Links  big screw 6 printed_v1 (Autodesk Fusion 360 design; units mm, degrees)
Autodesk Fusion 360 part; units mm, degrees
note: some values were not read from the file. Chosen so that the rebuilt part matches the saved one: which face or edge a step refers to. Set by a fixed rule: which sketch regions a step uses.
sketch "passive link sketch" plane through (0, 0, 0) normal (0, 0, 1) x (1, 0, 0)
  line L0 (-16.4533, 8) -> (-16.4533, -8) construction
  line L1 (16.4533, -8) -> (16.4533, 8) construction
  line L2 (16.4533, 8) -> (-16.4533, -8) construction
  line L3 (-16.4533, 8) -> (16.4533, -8) construction
  circle A0 centre (12.5, 0) radius 4.5
  circle A1 centre (12.5, 0) radius 2.975
  circle A2 centre (12.5, 0) radius 8
  line L4 (0, 8) -> (0, -15) construction
  line L5 (12.5, 8) -> (0, 8)
  line L6 (0, -8) -> (12.5, -8)
  line L7 (12.5, -8) -> (12.5, 8)
  line L8 (12.5, 8) -> (-12.5, -8) construction
  line L9 (-12.5, 8) -> (12.5, -8) construction
  line L10 (16.4533, 8) -> (0, 8) construction
  line L11 (-12.5, 8) -> (-16.4533, 8) construction
  line L12 (-16.4533, -8) -> (-12.5, -8) construction
  line L13 (0, -8) -> (16.4533, -8) construction
  line L14 (0, -8) -> (-16.4533, -8) construction
  line L15 (-12.5, -8) -> (-12.5, 8)
  line L16 (-16.4533, 8) -> (0, 8) construction
  circle A3 centre (-12.5, 0) radius 8
  circle A4 centre (-12.5, 0) radius 2.975
  circle A5 centre (-12.5, 0) radius 4.5
  line L17 (0, -8) -> (-12.5, -8)
  line L18 (-12.5, 8) -> (0, 8)
  dimension "d2" = 16
  dimension "d3" = 9
  dimension "d4" = 5.95
  dimension "d5" = 16
  dimension "d6" = 12.5
  dimension "d7" = 25
  constraint horizontal L10
  constraint perpendicular L0 L10
  constraint parallel L10 L12
  constraint parallel L0 L1
  constraint coincident L2 origin
  constraint coincident L3 origin
  constraint concentric A0 A1
  constraint concentric A0 A2
  constraint perpendicular L4 L12
  constraint horizontal origin A0.centre
  constraint horizontal L5
  constraint parallel L5 L6
  constraint coincident A2 L5.start
  constraint coincident L8 origin
  constraint coincident L9 origin
  constraint collinear L10 L11
  constraint coincident L4 L6.start
  constraint collinear L12 L13
  constraint symmetric L1.end L4 L0.start
  constraint symmetric L1.start L4 L0.end
  constraint symmetric A0 L4 A5
  constraint symmetric A1 L4 A4
  constraint symmetric A2 L4 A3
  constraint symmetric L4 L5.start L9.start
  constraint symmetric L4 L6.end L8.end
  constraint symmetric L4 L5.end L10.end
  constraint symmetric L4 L6.start L13.start
  constraint perpendicular L15 L18
  constraint coincident L4 origin
  measures "d2" distance of L0.start L0.end
  measures "d3" diameter of A0
  measures "d4" diameter of A1
  measures "d5" diameter of A2
  measures "d6" distance of origin A0.centre
  measures "d7" distance of L8.end L6.end
extrude "base" add sketch "passive link sketch" along normal mid plane 4 contours A0 A1 L7 | A0 A2 L7 | A2 L5 L6 A3 L17 L18 | L15 A3 A5 | L15 A4 A5 picked at (11.6865, -3.8972) picked at (12.1026, -6.8035) picked at (-12.1205, 6.8062) picked at (-11.7228, 3.9055) makes body 1
extrude "l  big cyl" add sketch "passive link sketch" along normal blind 5 and the other way blind 6 separate body contours L15 A3 A5 | L15 A3 A5 | L15 A4 A5 | L15 A4 A5 makes body 2
fillet "Fillet13" radius 3 1 edges at (-19.9586, 2.8929, -6) on bodies 2
fillet "Fillet9" radius 0.3 1 edges at (-19.9586, -2.8929, 5) on bodies 2
extrude "Extrude8" add sketch "passive link sketch" along normal blind 5 and the other way blind 7 separate body contours L15 A4 A5 | L15 A4 A5 makes body 3
fillet "Fillet14" radius 0.3 1 edges at (-16.6955, 1.6273, -7) on bodies 3
sketch "Square nut hole" plane through (0, 0, 5) normal (0, 0, 1) x (1, 0, 0)
  circle A0 centre (-12.5, 0) radius 2.975
  line L0 (-18, 5.5) -> (-7, 5.5)
  line L1 (-7, 5.5) -> (-7, -5.5)
  line L2 (-7, -5.5) -> (-18, -5.5)
  line L3 (-18, -5.5) -> (-18, 5.5)
  line L4 (-18, 5.5) -> (-7, -5.5) construction
  line L5 (-7, 5.5) -> (-18, -5.5) construction
  circle A1 centre (-12.5, 0) radius 7.7
  point P0 (-12.5, 0)
  dimension "d148" = 11
  dimension "d149" = 11
  constraint horizontal L0
  constraint perpendicular L0 L1
  constraint parallel L0 L2
  constraint parallel L1 L3
  constraint coincident L4 P0
  constraint coincident L5 P0
  constraint coincident P0 A0.centre
  measures "d148" distance of L1.end L2.end
  measures "d149" distance of L0.end L1.end
extrude "Extrude17" cut sketch "Square nut hole" against normal blind 4 contours L0 L3 A1 | L0 L1 L2 L3 A1 | L0 L1 A1 | L2 L3 A1 | L1 L2 A1 bodies 2 3
mirror "Mirror1" about plane through (0, 0, 0) normal (1, 0, 0) of bodies 2 3 makes body 4 at (4.5398, 0.7965, -0.4333) makes body 5 at (8.0224, -0.4481, -4.1333)
mirror "Mirror2" about plane through (0, 0, 0) normal (0, 0, 1) of bodies 4 5 makes body 6 at (4.5398, 0.7965, 0.4333) makes body 7 at (8.0224, -0.4481, 4.1333)
delete_body "RemoveBody1" bodies 4
delete_body "RemoveBody2" bodies 5
sketch "motorLinkSketch" plane through (0, 0, 0) normal (0, 0, 1) x (-1, 0, 0) in component "MotorLinkComponent"
  line L0 (12.5, -8) -> (12.5, 8)
  line L1 (0, 8) -> (0, -15) construction
  circle A0 centre (12.5, 0) radius 8
  circle A1 centre (12.5, 0) radius 2.975
  circle A2 centre (12.5, 0) radius 4.5
  circle A3 centre (-12.5, 0) radius 2.55
  circle A4 centre (-12.5, 0) radius 8
  line L2 (12.5, 8) -> (-12.5, 8)
  line L3 (12.5, -8) -> (-12.5, -8)
  line L4 (-14.4, -1.7007) -> (-14.4, 1.7007)
  line L5 (-12.5, -8) -> (-12.5, 8)
  line L6 (-9.95, -3.9402) -> (-9.95, 0.0066) construction
  point P0 (-12.5, 0.7805)
  dimension "d215" = 9
  dimension "d216" = 5.95
  dimension "d217" = 16
  dimension "d218" = 12.5
  dimension "d222" = 16
  dimension "d223" = 5.1
  dimension "d261" = 25
  dimension "d262" = 4.45
  constraint concentric A1 A2
  constraint concentric A0 A2
  constraint horizontal origin A0.centre
  constraint coincident L0.end A0
  constraint coincident origin L1
  constraint coincident A4 L2.end
  constraint tangent A4 L2
  constraint perpendicular L0 L2
  constraint coincident A4 L3.end
  constraint tangent A4 L3
  constraint perpendicular L0 L3
  constraint horizontal L3
  constraint coincident A3 L4.end
  constraint vertical L4
  constraint perpendicular L2 L5
  constraint coincident A3.centre L5
  constraint coincident A3 L4.start
  constraint concentric A3 A4
  constraint vertical L6
  constraint tangent A3 L6
  measures "d215" diameter of A2
  measures "d216" diameter of A1
  measures "d217" diameter of A0
  measures "d218" distance of origin A0.centre
  measures "d222" diameter of A4
  measures "d223" diameter of A3
  measures "d261" distance of A0.centre A3.centre
  measures "d262" distance of L4 L6.start
extrude "Extrude13" add sketch "motorLinkSketch" along normal mid plane 4 separate body contours L0 A0 A2 | A0 A4 L2 L3 | L0 A1 A2 | A3 A4 L5 picked at (6.4092, -3.0576) picked at (10.9768, -3.6783) picked at (-6.3438, -0.3795) makes body 8 in component "MotorLinkComponent"
extrude "Extrude14" add sketch "motorLinkSketch" along normal blind 5 and the other way blind 6 separate body contours L0 A0 A2 | L0 A0 A2 | L0 A1 A2 | L0 A1 A2 makes body 9 in component "MotorLinkComponent"
extrude "Extrude15" add sketch "motorLinkSketch" along normal blind -5 and the other way blind 7 contours L0 A1 A2 | L0 A1 A2 bodies 9 in component "MotorLinkComponent"
fillet "Fillet5" radius 3 1 edges at (-5.0414, -2.8929, -6) on bodies 9 in component "MotorLinkComponent"
fillet "Fillet6" radius 0.3 1 edges at (-8.3045, -1.6273, -7) on bodies 9 in component "MotorLinkComponent"
fillet "Fillet7" radius 0.3 1 edges at (-5.0414, 2.8929, 5) on bodies 9 in component "MotorLinkComponent"
extrude "Extrude16" add sketch "motorLinkSketch" along normal blind 9 and the other way blind 2 separate body contours A3 A4 L5 | A3 A4 L5 | A3 L4 makes body 10 in component "MotorLinkComponent"
fillet "Fillet8" radius 0.3 1 edges at (19.9586, 2.8929, 9) on bodies 10 in component "MotorLinkComponent"
fillet "Fillet9'" radius 0.3 3 edges at (0, 8, -2) (19.9586, -2.8929, -2) (0, -8, -2) on bodies 8 10 in component "MotorLinkComponent"
fillet "Fillet10" radius 0.3 1 edges at (0, 8, 2) on bodies 8 in component "MotorLinkComponent"
fillet "Fillet11" radius 0.3 1 edges at (0, -8, 2) on bodies 8 in component "MotorLinkComponent"
fillet "Fillet12" radius 0.3 2 edges at (9.95, 0, 9) (14.4, 0, 9) on bodies 10 in component "MotorLinkComponent"
sketch "Sketch7" plane through (10, 0, 5) normal (0, 0, 1) x (-1, 0, 0)
  circle A0 centre (-27.5, 0) radius 2.975
  circle A1 centre (-27.5, 0) radius 7.7
  line L0 (-22, -5.5) -> (-33, -5.5)
  line L1 (-33, -5.5) -> (-33, 5.5)
  line L2 (-33, 5.5) -> (-22, 5.5)
  line L3 (-22, 5.5) -> (-22, -5.5)
  line L4 (-22, -5.5) -> (-33, 5.5) construction
  line L5 (-33, -5.5) -> (-22, 5.5) construction
  point P0 (-27.5, 0)
  dimension "d263" = 11
  dimension "d264" = 11
  constraint horizontal L0
  constraint perpendicular L0 L1
  constraint parallel L0 L2
  constraint parallel L1 L3
  constraint coincident L4 P0
  constraint coincident L5 P0
  constraint coincident P0 A0.centre
  measures "d263" distance of L1.end L2.end
  measures "d264" distance of L0.end L1.end
extrude "Extrude17'" cut sketch "Sketch7" against normal blind 5 contours A1 L0 L1 L2 L3 sketch seen with x (1, 0, 0) y (0, 1, 0) z (0, 0, 1) at (-50, 0, 0) bodies 8 9 in component "MotorLinkComponent"
component "MotorLinkComponent" placed x (1, 0, 0) y (0, 1, 0) z (0, 0, 1) at (50, 0, 0)
equation "d2 = bigBarrelDiam"
equation "d3 = restShoulderDiam"
equation "d4 = screwHoleDiam"
equation "d5 = bigBarrelDiam"
equation "d8 = rectHeight / 2"
equation "d16 = nutSideHeight"
equation "d22 = nutSideHeight"
equation "d24 = maxScrewSideHeight"
equation "d25 = 0.0 °"
equation "d52 = maxScrewSideHeight - 1 mm"
equation "d53 = 0.0 °"
equation "rectHeight = 4 mm"
equation "bigBarrelDiam = 16 mm"
equation "screwHoleDiam = 5.95 mm"
equation "shaftDiameter = 5.1 mm"
equation "rectLen = 25 mm"
equation "d134 = -nutDepth"
equation "d148 = nutDimesion"
equation "d149 = nutDimesion"
equation "d151 = smallFillet"
equation "restShoulderDiam = 9 mm"
equation "nutSideHeight = 5 mm"
equation "maxScrewSideHeight = 7 mm"
equation "d206 = bigFillet"
equation "nutDepth = 4 mm"
equation "d209 = smallFillet"
equation "shaftNotchDelta = 4.45 mm"
equation "d215 = restShoulderDiam"
equation "d216 = screwHoleDiam"
equation "d217 = bigBarrelDiam"
equation "d218 = rectLen / 2"
equation "d222 = bigBarrelDiam"
equation "d223 = shaftDiameter"
equation "d228 = rectHeight / 2"
equation "d230 = nutSideHeight"
equation "d232 = maxScrewSideHeight - 1 mm"
equation "d233 = 0.0 °"
equation "d234 = -nutSideHeight"
equation "d236 = maxScrewSideHeight"
equation "d237 = 0.0 °"
equation "bigFillet = 3 mm"
equation "smallFillet = 0.3 mm"
equation "d241 = bigFillet"
equation "d243 = smallFillet"
equation "d245 = smallFillet"
equation "shaftHeightFromBottom = 7 mm"
equation "d247 = rectHeight / 2 + shaftHeightFromBottom"
equation "d250 = 0.0 °"
equation "d252 = smallFillet"
equation "d254 = smallFillet"
equation "d256 = smallFillet"
equation "d258 = smallFillet"
equation "d260 = smallFillet"
equation "d261 = rectLen"
equation "d262 = shaftNotchDelta"
equation "d263 = nutDimesion"
equation "d264 = nutDimesion"
equation "nutDimesion = 11 mm"
equation "d266 = -nutSideHeight"
named bodies: "big barrel", "screwHole", "big barrel (1)", "screwHole (1)", "big barrel (1) (1)", "screwHole (1) (1)", "cuboid", "link part", "motor part"
